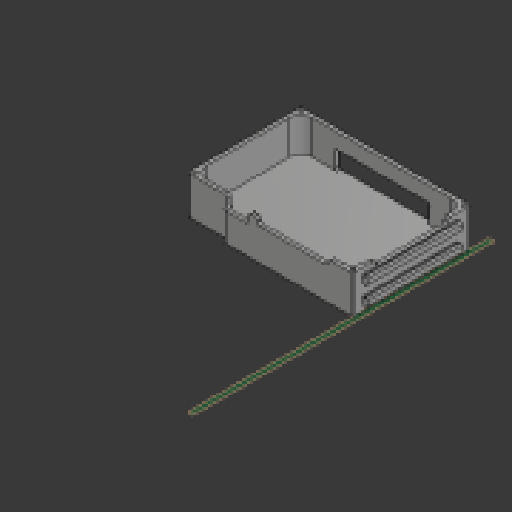
# Autodesk Inventor part: Back_Case
Saved by Autodesk Inventor 2023 (Build 270158000, 158)
## iProperties
Created: 2023-01-07
Part Number: Back_Case
Material: Generic
Document SubType Name: Modeling
Designer: alber
Density: 1 g/cm^3
Appearance: Smooth - Medium Gray
Author: alber
Autodesk Inventor part; units mm, degrees
ref_plane "YZ Plane" through (0, 0, 0) normal (1, 0, 0) x (0, 1, 0)
ref_plane "XZ Plane" through (0, 0, 0) normal (0, 1, 0) x (-1, 0, 0)
ref_plane "XY Plane" through (0, 0, 0) normal (0, 0, 1) x (1, 0, 0)
ref_plane "Work Plane1" through (64.9475, 0, 227.1619) normal (0, -1, 0) x (0, 0, 1)
sketch "Sketch1" plane through (64.9475, 0, 227.1619) normal (0, -1, 0) x (0, 0, 1)
  line L0 (-165, 215) -> (-165, 20) projected
  line L1 (-290, 20) -> (-165, 20)
  line L2 (-165, 20) -> (-165, 200)
  line L3 (-165, 200) -> (-290, 200)
  line L4 (-290, 200) -> (-290, 20)
  line L5 (0.8, 269) -> (0.8, 158) projected
  arc A0 (-0.2, 157) -> (0.8, 158) centre (-0.2, 158) ccw projected
  line L6 (-0.2, 157) -> (-164.2, 157) projected
  arc A1 (-165.2, 158) -> (-164.2, 157) centre (-164.2, 158) ccw projected
  line L7 (-165.2, 158) -> (-165.2, 269) projected
  arc A2 (-164.2, 270) -> (-165.2, 269) centre (-164.2, 269) ccw projected
  line L8 (-164.2, 270) -> (-126.2, 270) projected
  arc A3 (-125.2, 269) -> (-126.2, 270) centre (-126.2, 269) ccw projected
  line L9 (-125.2, 269) -> (-125.2, 267) projected
  arc A4 (-125.2, 267) -> (-124.2, 266) centre (-124.2, 267) ccw projected
  line L10 (-124.2, 266) -> (-116.2, 266) projected
  arc A5 (-116.2, 266) -> (-115.2, 267) centre (-116.2, 267) ccw projected
  line L11 (-115.2, 267) -> (-115.2, 269) projected
  arc A6 (-114.2, 270) -> (-115.2, 269) centre (-114.2, 269) ccw projected
  line L12 (-114.2, 270) -> (-0.2, 270) projected
  arc A7 (0.8, 269) -> (-0.2, 270) centre (-0.2, 269) ccw projected
  circle A8 centre (-38.2, 210.5) radius 5.1429 projected
  arc A9 (-20.2629, 212.0039) -> (-36.7039, 228.4377) centre (-38.2, 210.5) ccw projected
  line L13 (-36.7039, 228.4377) -> (-36.7039, 223.2698) projected
  arc A10 (-25.4311, 212.0039) -> (-36.7039, 223.2698) centre (-38.2, 210.5) ccw projected
  line L14 (-25.4311, 212.0039) -> (-20.2629, 212.0039) projected
  arc A11 (-28.0248, 212.0039) -> (-36.7039, 220.6763) centre (-38.2, 210.5) ccw projected
  line L15 (-36.7039, 220.6763) -> (-36.7039, 218.0678) projected
  arc A12 (-30.6322, 211.9961) -> (-36.7039, 218.0678) centre (-38.2, 210.5) ccw projected
  line L16 (-30.6322, 211.9961) -> (-30.6322, 212.0039) projected
  line L17 (-30.6322, 212.0039) -> (-28.0248, 212.0039) projected
  line L18 (-39.7039, 223.2689) -> (-39.7039, 228.4371) projected
  arc A13 (-39.7039, 228.4371) -> (-56.1377, 211.9961) centre (-38.2, 210.5) ccw projected
  line L19 (-56.1377, 211.9961) -> (-50.9698, 211.9961) projected
  arc A14 (-39.7039, 223.2689) -> (-50.9698, 211.9961) centre (-38.2, 210.5) ccw projected
  line L20 (-39.7039, 218.0678) -> (-39.7039, 220.6752) projected
  arc A15 (-39.7039, 220.6752) -> (-48.3763, 211.9961) centre (-38.2, 210.5) ccw projected
  line L21 (-48.3763, 211.9961) -> (-45.7678, 211.9961) projected
  arc A16 (-39.6961, 218.0678) -> (-45.7678, 211.9961) centre (-38.2, 210.5) ccw projected
  line L22 (-39.6961, 218.0678) -> (-39.7039, 218.0678) projected
  line L23 (-50.9689, 208.9961) -> (-56.1371, 208.9961) projected
  arc A17 (-56.1371, 208.9961) -> (-39.6961, 192.5623) centre (-38.2, 210.5) ccw projected
  line L24 (-39.6961, 192.5623) -> (-39.6961, 197.7302) projected
  arc A18 (-50.9689, 208.9961) -> (-39.6961, 197.7302) centre (-38.2, 210.5) ccw projected
  line L25 (-45.7678, 208.9961) -> (-48.3752, 208.9961) projected
  arc A19 (-48.3752, 208.9961) -> (-39.6961, 200.3237) centre (-38.2, 210.5) ccw projected
  line L26 (-39.6961, 200.3237) -> (-39.6961, 202.9322) projected
  arc A20 (-45.7678, 209.0039) -> (-39.6961, 202.9322) centre (-38.2, 210.5) ccw projected
  line L27 (-45.7678, 209.0039) -> (-45.7678, 208.9961) projected
  arc A21 (-36.6961, 197.7311) -> (-25.4302, 209.0039) centre (-38.2, 210.5) ccw projected
  line L28 (-36.6961, 197.7311) -> (-36.6961, 192.5629) projected
  arc A22 (-36.6961, 192.5629) -> (-20.2623, 209.0039) centre (-38.2, 210.5) ccw projected
  line L29 (-20.2623, 209.0039) -> (-25.4302, 209.0039) projected
  line L30 (-36.6961, 202.9322) -> (-36.6961, 200.3248) projected
  arc A23 (-36.6961, 200.3248) -> (-28.0237, 209.0039) centre (-38.2, 210.5) ccw projected
  line L31 (-28.0237, 209.0039) -> (-30.6322, 209.0039) projected
  arc A24 (-36.7039, 202.9322) -> (-30.6322, 209.0039) centre (-38.2, 210.5) ccw projected
  line L32 (-36.7039, 202.9322) -> (-36.6961, 202.9322) projected
  arc A25 (-137, 209.9) -> (-133.4, 209.9) centre (-135.2, 209.9) ccw projected
  line L33 (-133.4, 209.9) -> (-133.4, 214.1) projected
  arc A26 (-133.4, 214.1) -> (-137, 214.1) centre (-135.2, 214.1) ccw projected
  line L34 (-137, 214.1) -> (-137, 209.9) projected
  circle A27 centre (-6.7, 162) radius 2.1 projected
  circle A28 centre (-6.7, 265) radius 2.1 projected
  point P0 (-227.1619, 64.9475)
  point P1 (-165, 200)
  point P2 (-132.7045, 157)
  point P3 (-165.2, 200)
  point P4 (-165, 157.4)
  dimension "d0" = 125
  dimension "d1" = 180
  constraints: 8 end point, 2 parallel, 1 collinear, 1 horizontal, 1 perpendicular
  measures "d0" distance of L3.end L2.end
  measures "d1" distance of L2.end L1.end
extrude "Extrusion1" add sketch "Sketch1" against normal blind 4 contours L0 A1 L7 L3 | L0 L1 L4 L3 L7 A1
sketch "Sketch2" plane through (64.9475, 4, 227.1619) normal (0, 1, 0) x (1, 0, 0)
  line L0 (-20, 165) -> (-20, 290) projected
  line L1 (-20, 290) -> (-200, 290) projected
  line L2 (-200, 290) -> (-200, 165) projected
  line L3 (-200, 165) -> (-20, 165) projected
  line L4 (-24, 169) -> (-24, 286)
  line L5 (-24, 286) -> (-196, 286)
  line L6 (-196, 286) -> (-196, 169)
  line L7 (-196, 169) -> (-24, 169)
  arc A0 (-157, 164.2) -> (-158, 165.2) centre (-158, 164.2) ccw
  line L8 (-157, 160.2816) -> (-157, 164.2)
  line L9 (-158, 165.2) -> (-196, 165.2)
  line L10 (-200, 165.2) -> (-269, 165.2)
  line L11 (-153, 164.2) -> (-153, 160.2816)
  point P0 (-64.9475, 227.1619)
  point P1 (-157.0033, 164.2816)
  dimension "d4" = 4
  constraints: 16 end point, 2 horizontal, 2 point on circle, 2 point on line, 1 centre point, 1 vertical, 11 other
ref_plane "Work Plane2" through (45.1475, 40, -62.8381) normal (0, 1, 0) x (0, 0, 1)
extrude "Extrusion2" add sketch "Sketch2" along normal up to surface (36 mm away)
sketch "Sketch3" plane through (44.9475, 0, -62.8381) normal (0, 0, -1) x (-1, 0, 0)
  line L0 (-25.1172, 40) -> (-14.8828, 40) projected
  arc A0 (-25.1172, 40) -> (-25.2586, 39.9414) centre (-25.1172, 39.8) ccw projected
  line L1 (-26.6586, 38.5414) -> (-25.2586, 39.9414) projected
  arc A1 (-26.6586, 38.5414) -> (-26.5172, 38.2) centre (-26.5172, 38.4) ccw projected
  line L2 (-26.5172, 38.2) -> (-24.7899, 38.2) projected
  line L3 (-24.7899, 36.2) -> (-24.7899, 38.2) projected
  line L4 (-26.9899, 34) -> (-24.7899, 36.2) projected
  line L5 (-29.5, 34) -> (-26.9899, 34) projected
  line L6 (-29.5, 34) -> (-30, 33.5) projected
  line L7 (-30, 33.5) -> (-30.5, 34) projected
  line L8 (-33.0101, 34) -> (-30.5, 34) projected
  line L9 (-35.2101, 36.2) -> (-33.0101, 34) projected
  line L10 (-35.2101, 38.2) -> (-35.2101, 36.2) projected
  line L11 (-35.2101, 38.2) -> (-33.4828, 38.2) projected
  arc A2 (-33.4828, 38.2) -> (-33.3414, 38.5414) centre (-33.4828, 38.4) ccw projected
  line L12 (-34.7414, 39.9414) -> (-33.3414, 38.5414) projected
  arc A3 (-34.7414, 39.9414) -> (-34.8828, 40) centre (-34.8828, 39.8) ccw projected
  line L13 (-39.8, 40) -> (-34.8828, 40) projected
  arc A4 (-39.8, 40) -> (-40, 39.8) centre (-39.8, 39.8) ccw projected
  line L14 (-40, 34.8828) -> (-40, 39.8) projected
  arc A5 (-40, 34.8828) -> (-39.9414, 34.7414) centre (-39.8, 34.8828) ccw projected
  line L15 (-38.5414, 33.3414) -> (-39.9414, 34.7414) projected
  arc A6 (-38.5414, 33.3414) -> (-38.2, 33.4828) centre (-38.4, 33.4828) ccw projected
  line L16 (-38.2, 33.4828) -> (-38.2, 35.2101) projected
  line L17 (-36.2, 35.2101) -> (-38.2, 35.2101) projected
  line L18 (-34, 33.0101) -> (-36.2, 35.2101) projected
  line L19 (-34, 30.5) -> (-34, 33.0101) projected
  line L20 (-34, 30.5) -> (-33.5, 30) projected
  line L21 (-33.5, 30) -> (-34, 29.5) projected
  line L22 (-34, 26.9899) -> (-34, 29.5) projected
  line L23 (-36.2, 24.7899) -> (-34, 26.9899) projected
  line L24 (-38.2, 24.7899) -> (-36.2, 24.7899) projected
  line L25 (-38.2, 24.7899) -> (-38.2, 26.5172) projected
  arc A7 (-38.2, 26.5172) -> (-38.5414, 26.6586) centre (-38.4, 26.5172) ccw projected
  line L26 (-39.9414, 25.2586) -> (-38.5414, 26.6586) projected
  arc A8 (-39.9414, 25.2586) -> (-40, 25.1172) centre (-39.8, 25.1172) ccw projected
  line L27 (-40, 14.8) -> (-40, 25.1172) projected
  line L28 (-38.2, 13) -> (-40, 14.8) projected
  line L29 (-38.2, 15.2101) -> (-38.2, 13) projected
  line L30 (-36.2, 15.2101) -> (-38.2, 15.2101) projected
  line L31 (-34, 13.0101) -> (-36.2, 15.2101) projected
  line L32 (-34, 10.5) -> (-34, 13.0101) projected
  line L33 (-33.5, 10) -> (-34, 10.5) projected
  line L34 (-34, 9.5) -> (-33.5, 10) projected
  line L35 (-34, 6.9899) -> (-34, 9.5) projected
  line L36 (-36.2, 4.7899) -> (-34, 6.9899) projected
  line L37 (-38.2, 4.7899) -> (-36.2, 4.7899) projected
  line L38 (-38.2, 7) -> (-38.2, 4.7899) projected
  line L39 (-40, 5.2) -> (-38.2, 7) projected
  line L40 (-40, 0) -> (-40, 5.2) projected
  line L41 (-34.8, 0) -> (-40, 0) projected
  line L42 (-33, 1.8) -> (-34.8, 0) projected
  line L43 (-35.2101, 1.8) -> (-33, 1.8) projected
  line L44 (-35.2101, 3.8) -> (-35.2101, 1.8) projected
  line L45 (-33.0101, 6) -> (-35.2101, 3.8) projected
  line L46 (-30.5, 6) -> (-33.0101, 6) projected
  line L47 (-30, 6.5) -> (-30.5, 6) projected
  line L48 (-29.5, 6) -> (-30, 6.5) projected
  line L49 (-26.9899, 6) -> (-29.5, 6) projected
  line L50 (-24.7899, 3.8) -> (-26.9899, 6) projected
  line L51 (-24.7899, 1.8) -> (-24.7899, 3.8) projected
  line L52 (-27, 1.8) -> (-24.7899, 1.8) projected
  line L53 (-25.2, 0) -> (-27, 1.8) projected
  line L54 (-14.8, 0) -> (-25.2, 0) projected
  line L55 (-13, 1.8) -> (-14.8, 0) projected
  line L56 (-15.2101, 1.8) -> (-13, 1.8) projected
  line L57 (-15.2101, 3.8) -> (-15.2101, 1.8) projected
  line L58 (-13.0101, 6) -> (-15.2101, 3.8) projected
  line L59 (-10.5, 6) -> (-13.0101, 6) projected
  line L60 (-10, 6.5) -> (-10.5, 6) projected
  line L61 (-9.5, 6) -> (-10, 6.5) projected
  line L62 (-6.9899, 6) -> (-9.5, 6) projected
  line L63 (-4.7899, 3.8) -> (-6.9899, 6) projected
  line L64 (-4.7899, 1.8) -> (-4.7899, 3.8) projected
  line L65 (-7, 1.8) -> (-4.7899, 1.8) projected
  line L66 (-5.2, 0) -> (-7, 1.8) projected
  line L67 (0, 0) -> (-5.2, 0) projected
  line L68 (0, 5.2) -> (0, 0) projected
  line L69 (-1.8, 7) -> (0, 5.2) projected
  line L70 (-1.8, 4.7899) -> (-1.8, 7) projected
  line L71 (-3.8, 4.7899) -> (-1.8, 4.7899) projected
  line L72 (-6, 6.9899) -> (-3.8, 4.7899) projected
  line L73 (-6, 9.5) -> (-6, 6.9899) projected
  line L74 (-6.5, 10) -> (-6, 9.5) projected
  line L75 (-6, 10.5) -> (-6.5, 10) projected
  line L76 (-6, 13.0101) -> (-6, 10.5) projected
  line L77 (-3.8, 15.2101) -> (-6, 13.0101) projected
  line L78 (-1.8, 15.2101) -> (-3.8, 15.2101) projected
  line L79 (-1.8, 13) -> (-1.8, 15.2101) projected
  line L80 (0, 14.8) -> (-1.8, 13) projected
  line L81 (0, 25.1172) -> (0, 14.8) projected
  arc A9 (0, 25.1172) -> (-0.0586, 25.2586) centre (-0.2, 25.1172) ccw projected
  line L82 (-1.4586, 26.6586) -> (-0.0586, 25.2586) projected
  arc A10 (-1.4586, 26.6586) -> (-1.8, 26.5172) centre (-1.6, 26.5172) ccw projected
  line L83 (-1.8, 26.5172) -> (-1.8, 24.7899) projected
  line L84 (-3.8, 24.7899) -> (-1.8, 24.7899) projected
  line L85 (-6, 26.9899) -> (-3.8, 24.7899) projected
  line L86 (-6, 29.5) -> (-6, 26.9899) projected
  line L87 (-6, 29.5) -> (-6.5, 30) projected
  line L88 (-6.5, 30) -> (-6, 30.5) projected
  line L89 (-6, 33.0101) -> (-6, 30.5) projected
  line L90 (-3.8, 35.2101) -> (-6, 33.0101) projected
  line L91 (-1.8, 35.2101) -> (-3.8, 35.2101) projected
  line L92 (-1.8, 35.2101) -> (-1.8, 33.4828) projected
  arc A11 (-1.8, 33.4828) -> (-1.4586, 33.3414) centre (-1.6, 33.4828) ccw projected
  line L93 (-0.0586, 34.7414) -> (-1.4586, 33.3414) projected
  arc A12 (-0.0586, 34.7414) -> (0, 34.8828) centre (-0.2, 34.8828) ccw projected
  line L94 (0, 39.8) -> (0, 34.8828) projected
  arc A13 (0, 39.8) -> (-0.2, 40) centre (-0.2, 39.8) ccw projected
  line L95 (-5.1172, 40) -> (-0.2, 40) projected
  arc A14 (-5.1172, 40) -> (-5.2586, 39.9414) centre (-5.1172, 39.8) ccw projected
  line L96 (-6.6586, 38.5414) -> (-5.2586, 39.9414) projected
  arc A15 (-6.6586, 38.5414) -> (-6.5172, 38.2) centre (-6.5172, 38.4) ccw projected
  line L97 (-6.5172, 38.2) -> (-4.7899, 38.2) projected
  line L98 (-4.7899, 36.2) -> (-4.7899, 38.2) projected
  line L99 (-6.9899, 34) -> (-4.7899, 36.2) projected
  line L100 (-9.5, 34) -> (-6.9899, 34) projected
  line L101 (-9.5, 34) -> (-10, 33.5) projected
  line L102 (-10, 33.5) -> (-10.5, 34) projected
  line L103 (-13.0101, 34) -> (-10.5, 34) projected
  line L104 (-15.2101, 36.2) -> (-13.0101, 34) projected
  line L105 (-15.2101, 38.2) -> (-15.2101, 36.2) projected
  line L106 (-15.2101, 38.2) -> (-13.4828, 38.2) projected
  arc A16 (-13.4828, 38.2) -> (-13.3414, 38.5414) centre (-13.4828, 38.4) ccw projected
  line L107 (-14.7414, 39.9414) -> (-13.3414, 38.5414) projected
  arc A17 (-14.7414, 39.9414) -> (-14.8828, 40) centre (-14.8828, 39.8) ccw projected
  circle A18 centre (-30, 30) radius 3 projected
  circle A19 centre (-10, 10) radius 3 projected
  circle A20 centre (-10, 30) radius 2.5 projected
  circle A21 centre (-30, 10) radius 2.5 projected
  line L108 (-13.0101, 14) -> (-14, 13.0101) projected
  line L109 (-14, 10.5) -> (-14, 13.0101) projected
  line L110 (-13.5, 10) -> (-14, 10.5) projected
  line L111 (-14, 9.5) -> (-13.5, 10) projected
  line L112 (-14, 6.9899) -> (-14, 9.5) projected
  line L113 (-16.2, 4.7899) -> (-14, 6.9899) projected
  line L114 (-23.8, 4.7899) -> (-16.2, 4.7899) projected
  line L115 (-26, 6.9899) -> (-23.8, 4.7899) projected
  line L116 (-26, 9.5) -> (-26, 6.9899) projected
  line L117 (-26.5, 10) -> (-26, 9.5) projected
  line L118 (-26, 10.5) -> (-26.5, 10) projected
  line L119 (-26, 13.0101) -> (-26, 10.5) projected
  line L120 (-26, 13.0101) -> (-26.9899, 14) projected
  line L121 (-29.5, 14) -> (-26.9899, 14) projected
  line L122 (-30, 13.5) -> (-29.5, 14) projected
  line L123 (-30.5, 14) -> (-30, 13.5) projected
  line L124 (-33.0101, 14) -> (-30.5, 14) projected
  line L125 (-35.2101, 16.2) -> (-33.0101, 14) projected
  line L126 (-38.2, 16.2) -> (-35.2101, 16.2) projected
  line L127 (-38.2, 23.8) -> (-38.2, 16.2) projected
  line L128 (-35.2101, 23.8) -> (-38.2, 23.8) projected
  line L129 (-33.0101, 26) -> (-35.2101, 23.8) projected
  line L130 (-30.5, 26) -> (-33.0101, 26) projected
  line L131 (-30.5, 26) -> (-30, 26.5) projected
  line L132 (-30, 26.5) -> (-29.5, 26) projected
  line L133 (-26.9899, 26) -> (-29.5, 26) projected
  line L134 (-26.9899, 26) -> (-26, 26.9899) projected
  line L135 (-26, 29.5) -> (-26, 26.9899) projected
  line L136 (-26, 29.5) -> (-26.5, 30) projected
  line L137 (-26.5, 30) -> (-26, 30.5) projected
  line L138 (-26, 33.0101) -> (-26, 30.5) projected
  line L139 (-23.8, 35.2101) -> (-26, 33.0101) projected
  line L140 (-16.2, 35.2101) -> (-23.8, 35.2101) projected
  line L141 (-14, 33.0101) -> (-16.2, 35.2101) projected
  line L142 (-14, 30.5) -> (-14, 33.0101) projected
  line L143 (-14, 30.5) -> (-13.5, 30) projected
  line L144 (-13.5, 30) -> (-14, 29.5) projected
  line L145 (-14, 26.9899) -> (-14, 29.5) projected
  line L146 (-14, 26.9899) -> (-13.0101, 26) projected
  line L147 (-10.5, 26) -> (-13.0101, 26) projected
  line L148 (-10.5, 26) -> (-10, 26.5) projected
  line L149 (-10, 26.5) -> (-9.5, 26) projected
  line L150 (-6.9899, 26) -> (-9.5, 26) projected
  line L151 (-4.7899, 23.8) -> (-6.9899, 26) projected
  line L152 (-1.8, 23.8) -> (-4.7899, 23.8) projected
  line L153 (-1.8, 16.2) -> (-1.8, 23.8) projected
  line L154 (-4.7899, 16.2) -> (-1.8, 16.2) projected
  line L155 (-6.9899, 14) -> (-4.7899, 16.2) projected
  line L156 (-9.5, 14) -> (-6.9899, 14) projected
  line L157 (-10, 13.5) -> (-9.5, 14) projected
  line L158 (-10.5, 14) -> (-10, 13.5) projected
  line L159 (-13.0101, 14) -> (-10.5, 14) projected
  line L160 (0, 0) -> (0, 40) projected
  line L161 (-5.6, 32.8444) -> (-5.6, 30.3343)
  line L162 (-5.6, 30.3343) -> (-5.9343, 30)
  line L163 (-5.9343, 30) -> (-5.6, 29.6657)
  line L164 (-5.6, 29.6657) -> (-5.6, 27.1556)
  line L165 (-5.6, 27.1556) -> (-3.6343, 25.1899)
  line L166 (-3.6343, 25.1899) -> (-2.2, 25.1899)
  line L167 (-2.2, 25.1899) -> (-2.2, 26.5172)
  arc A22 (-1.1757, 26.9414) -> (-2.2, 26.5172) centre (-1.6, 26.5172) ccw
  line L168 (-1.1757, 26.9414) -> (0.2243, 25.5414)
  arc A23 (0.4, 25.1172) -> (0.2243, 25.5414) centre (-0.2, 25.1172) ccw
  line L169 (0.4, 25.1172) -> (0.4, 14.6343)
  line L170 (0.4, 14.6343) -> (-1.1757, 13.0586)
  line L171 (-2.2, 13.4828) -> (-2.2, 14.8101)
  line L172 (-2.2, 14.8101) -> (-3.6343, 14.8101)
  line L173 (-3.6343, 14.8101) -> (-5.6, 12.8444)
  line L174 (-5.6, 12.8444) -> (-5.6, 10.3343)
  line L175 (-5.6, 10.3343) -> (-5.9343, 10)
  line L176 (-5.9343, 10) -> (-5.6, 9.6657)
  line L177 (-5.6, 9.6657) -> (-5.6, 7.1556)
  line L178 (-5.6, 7.1556) -> (-3.6343, 5.1899)
  line L179 (-3.6343, 5.1899) -> (-2.2, 5.1899)
  line L180 (-2.2, 5.1899) -> (-2.2, 6.5172)
  line L181 (-1.1757, 6.9414) -> (0.4, 5.3657)
  line L182 (0.4, 5.3657) -> (0.4, -0.4)
  line L183 (0.4, -0.4) -> (-5.3657, -0.4)
  line L184 (-5.3657, -0.4) -> (-7.9657, 2.2)
  line L185 (-7.9657, 2.2) -> (-5.1899, 2.2)
  line L186 (-5.1899, 2.2) -> (-5.1899, 3.6343)
  line L187 (-5.1899, 3.6343) -> (-7.1556, 5.6)
  line L188 (-7.1556, 5.6) -> (-9.6657, 5.6)
  line L189 (-9.6657, 5.6) -> (-10, 5.9343)
  line L190 (-10, 5.9343) -> (-10.3343, 5.6)
  line L191 (-10.3343, 5.6) -> (-12.8444, 5.6)
  line L192 (-12.8444, 5.6) -> (-14.8101, 3.6343)
  line L193 (-14.8101, 3.6343) -> (-14.8101, 2.2)
  line L194 (-14.8101, 2.2) -> (-12.0343, 2.2)
  line L195 (-12.0343, 2.2) -> (-14.6343, -0.4)
  line L196 (-14.6343, -0.4) -> (-25.3657, -0.4)
  line L197 (-25.3657, -0.4) -> (-27.9657, 2.2)
  line L198 (-27.9657, 2.2) -> (-25.1899, 2.2)
  line L199 (-25.1899, 2.2) -> (-25.1899, 3.6343)
  line L200 (-25.1899, 3.6343) -> (-27.1556, 5.6)
  line L201 (-27.1556, 5.6) -> (-29.6657, 5.6)
  line L202 (-29.6657, 5.6) -> (-30, 5.9343)
  line L203 (-30, 5.9343) -> (-30.3343, 5.6)
  line L204 (-30.3343, 5.6) -> (-32.8444, 5.6)
  line L205 (-32.8444, 5.6) -> (-34.8101, 3.6343)
  line L206 (-34.8101, 3.6343) -> (-34.8101, 2.2)
  line L207 (-34.8101, 2.2) -> (-32.0343, 2.2)
  line L208 (-32.0343, 2.2) -> (-34.6343, -0.4)
  line L209 (-34.6343, -0.4) -> (-40.4, -0.4)
  line L210 (-40.4, -0.4) -> (-40.4, 5.3657)
  line L211 (-40.4, 5.3657) -> (-37.8, 7.9657)
  line L212 (-37.8, 7.9657) -> (-37.8, 5.1899)
  line L213 (-37.8, 5.1899) -> (-36.3657, 5.1899)
  line L214 (-36.3657, 5.1899) -> (-34.4, 7.1556)
  line L215 (-34.4, 7.1556) -> (-34.4, 9.6657)
  line L216 (-34.4, 9.6657) -> (-34.0657, 10)
  line L217 (-34.0657, 10) -> (-34.4, 10.3343)
  line L218 (-34.4, 10.3343) -> (-34.4, 12.8444)
  line L219 (-34.4, 12.8444) -> (-36.3657, 14.8101)
  line L220 (-36.3657, 14.8101) -> (-37.8, 14.8101)
  line L221 (-37.8, 14.8101) -> (-37.8, 12.0343)
  line L222 (-37.8, 12.0343) -> (-40.4, 14.6343)
  line L223 (-40.4, 14.6343) -> (-40.4, 25.1172)
  arc A24 (-40.2243, 25.5414) -> (-40.4, 25.1172) centre (-39.8, 25.1172) ccw
  line L224 (-40.2243, 25.5414) -> (-38.8243, 26.9414)
  arc A25 (-37.8, 26.5172) -> (-38.8243, 26.9414) centre (-38.4, 26.5172) ccw
  line L225 (-37.8, 26.5172) -> (-37.8, 25.1899)
  line L226 (-37.8, 25.1899) -> (-36.3657, 25.1899)
  line L227 (-36.3657, 25.1899) -> (-34.4, 27.1556)
  line L228 (-34.4, 27.1556) -> (-34.4, 29.6657)
  line L229 (-34.4, 29.6657) -> (-34.0657, 30)
  line L230 (-34.0657, 30) -> (-34.4, 30.3343)
  line L231 (-34.4, 30.3343) -> (-34.4, 32.8444)
  line L232 (-34.4, 32.8444) -> (-36.3657, 34.8101)
  line L233 (-36.3657, 34.8101) -> (-37.8, 34.8101)
  line L234 (-37.8, 34.8101) -> (-37.8, 33.4828)
  arc A26 (-38.8243, 33.0586) -> (-37.8, 33.4828) centre (-38.4, 33.4828) ccw
  line L235 (-38.8243, 33.0586) -> (-40.2243, 34.4586)
  arc A27 (-40.4, 34.8828) -> (-40.2243, 34.4586) centre (-39.8, 34.8828) ccw
  line L236 (-40.4, 34.8828) -> (-40.4, 39.8)
  arc A28 (-39.8, 40.4) -> (-40.4, 39.8) centre (-39.8, 39.8) ccw
  line L237 (-39.8, 40.4) -> (-34.8828, 40.4)
  arc A29 (-34.4586, 40.2243) -> (-34.8828, 40.4) centre (-34.8828, 39.8) ccw
  line L238 (-34.4586, 40.2243) -> (-33.0586, 38.8243)
  arc A30 (-33.4828, 37.8) -> (-33.0586, 38.8243) centre (-33.4828, 38.4) ccw
  line L239 (-33.4828, 37.8) -> (-34.8101, 37.8)
  line L240 (-34.8101, 37.8) -> (-34.8101, 36.3657)
  line L241 (-34.8101, 36.3657) -> (-32.8444, 34.4)
  line L242 (-32.8444, 34.4) -> (-30.3343, 34.4)
  line L243 (-30.3343, 34.4) -> (-30, 34.0657)
  line L244 (-30, 34.0657) -> (-29.6657, 34.4)
  line L245 (-29.6657, 34.4) -> (-27.1556, 34.4)
  line L246 (-27.1556, 34.4) -> (-25.1899, 36.3657)
  line L247 (-25.1899, 36.3657) -> (-25.1899, 37.8)
  line L248 (-25.1899, 37.8) -> (-26.5172, 37.8)
  arc A31 (-26.9414, 38.8243) -> (-26.5172, 37.8) centre (-26.5172, 38.4) ccw
  line L249 (-26.9414, 38.8243) -> (-25.5414, 40.2243)
  arc A32 (-25.1172, 40.4) -> (-25.5414, 40.2243) centre (-25.1172, 39.8) ccw
  line L250 (-25.1172, 40.4) -> (-14.8828, 40.4)
  arc A33 (-14.4586, 40.2243) -> (-14.8828, 40.4) centre (-14.8828, 39.8) ccw
  line L251 (-14.4586, 40.2243) -> (-13.0586, 38.8243)
  arc A34 (-13.4828, 37.8) -> (-13.0586, 38.8243) centre (-13.4828, 38.4) ccw
  line L252 (-13.4828, 37.8) -> (-14.8101, 37.8)
  line L253 (-14.8101, 37.8) -> (-14.8101, 36.3657)
  line L254 (-14.8101, 36.3657) -> (-12.8444, 34.4)
  line L255 (-12.8444, 34.4) -> (-10.3343, 34.4)
  line L256 (-10.3343, 34.4) -> (-10, 34.0657)
  line L257 (-10, 34.0657) -> (-9.6657, 34.4)
  line L258 (-9.6657, 34.4) -> (-7.1556, 34.4)
  line L259 (-7.1556, 34.4) -> (-5.1899, 36.3657)
  line L260 (-5.1899, 36.3657) -> (-5.1899, 37.8)
  line L261 (-5.1899, 37.8) -> (-6.5172, 37.8)
  arc A35 (-6.9414, 38.8243) -> (-6.5172, 37.8) centre (-6.5172, 38.4) ccw
  line L262 (-6.9414, 38.8243) -> (-5.5414, 40.2243)
  arc A36 (-5.1172, 40.4) -> (-5.5414, 40.2243) centre (-5.1172, 39.8) ccw
  line L263 (-5.1172, 40.4) -> (-0.2, 40.4)
  arc A37 (0.4, 39.8) -> (-0.2, 40.4) centre (-0.2, 39.8) ccw
  line L264 (0.4, 39.8) -> (0.4, 34.8828)
  arc A38 (0.2243, 34.4586) -> (0.4, 34.8828) centre (-0.2, 34.8828) ccw
  line L265 (0.2243, 34.4586) -> (-1.1757, 33.0586)
  arc A39 (-2.2, 33.4828) -> (-1.1757, 33.0586) centre (-1.6, 33.4828) ccw
  line L266 (-2.2, 33.4828) -> (-2.2, 34.8101)
  line L267 (-2.2, 34.8101) -> (-3.6343, 34.8101)
  line L268 (-3.6343, 34.8101) -> (-5.6, 32.8444)
  arc A40 (-2.2, 13.4828) -> (-1.1757, 13.0586) centre (-1.6, 13.4828) ccw
  arc A41 (-1.1757, 6.9414) -> (-2.2, 6.5172) centre (-1.6, 6.5172) ccw
  line L269 (-5.6, 10.3343) -> (-5.6, 9.6657)
  line L270 (-5.6, 30.3343) -> (-5.6, 29.6657)
  point P0 (44.9475, 0)
  point P1 (0, 25.7657)
  point P2 (0, 34.2343)
  point P3 (0, 5.7657)
  point P4 (0, 14.2343)
  point P5 (0, 4)
  dimension "d7" = 0.4
  dimension "d8" = 0.6
  dimension "d9" = 0.6
  constraints: 220 end point, 40 point on circle, 20 centre point, 4 tangent, 1 collinear, 1 vertical, 125 other
  measures "d7" distance between parallel lines of L90 L268
  measures "d8" radius of A40
  measures "d9" radius of A41
extrude "Extrusion3" add sketch "Sketch3" against normal blind 115 contours L160 L168 A22 L167 L166 L165 L164 L270 L161 L268 L267 L266 A39 L265 | L160 L181 A41 L180 L179 L178 L177 L269 L174 L173 L172 L171 A40 L170
sketch "Sketch4" plane through (44.9475, 0, -62.8381) normal (0, 0, -1) x (-1, 0, 0)
  line L0 (180, 0) -> (0, 0) projected
  line L1 (180, 0) -> (180, 40) projected
  line L2 (0, 34.2343) -> (0, 40) projected
  line L3 (0, 25.7657) -> (0, 34.2343) projected
  line L4 (0, 5.7657) -> (0, 34.2343)
  line L5 (180, 40) -> (0, 40) projected
  line L6 (0, 34.2343) -> (-1.1757, 33.0586) projected
  arc A0 (-2.2, 33.4828) -> (-1.1757, 33.0586) centre (-1.6, 33.4828) ccw projected
  line L7 (-2.2, 33.4828) -> (-2.2, 34.8101) projected
  line L8 (-2.2, 34.8101) -> (-3.6343, 34.8101) projected
  line L9 (-3.6343, 34.8101) -> (-5.6, 32.8444) projected
  line L10 (-5.6, 32.8444) -> (-5.6, 27.1556) projected
  line L11 (-5.6, 27.1556) -> (-3.6343, 25.1899) projected
  line L12 (-3.6343, 25.1899) -> (-2.2, 25.1899) projected
  line L13 (-2.2, 25.1899) -> (-2.2, 26.5172) projected
  arc A1 (-1.1757, 26.9414) -> (-2.2, 26.5172) centre (-1.6, 26.5172) ccw projected
  line L14 (-1.1757, 26.9414) -> (0, 25.7657) projected
  line L15 (0, 14.2343) -> (0, 25.7657) projected
  line L16 (0, 14.2343) -> (-1.1757, 13.0586) projected
  arc A2 (-2.2, 13.4828) -> (-1.1757, 13.0586) centre (-1.6, 13.4828) ccw projected
  line L17 (-2.2, 13.4828) -> (-2.2, 14.8101) projected
  line L18 (-2.2, 14.8101) -> (-3.6343, 14.8101) projected
  line L19 (-3.6343, 14.8101) -> (-5.6, 12.8444) projected
  line L20 (-5.6, 12.8444) -> (-5.6, 7.1556) projected
  line L21 (-5.6, 7.1556) -> (-3.6343, 5.1899) projected
  line L22 (-3.6343, 5.1899) -> (-2.2, 5.1899) projected
  line L23 (-2.2, 5.1899) -> (-2.2, 6.5172) projected
  arc A3 (-1.1757, 6.9414) -> (-2.2, 6.5172) centre (-1.6, 6.5172) ccw projected
  line L24 (-1.1757, 6.9414) -> (0, 5.7657) projected
  line L25 (0, 0) -> (0, 5.7657) projected
  point P0 (44.9475, 0)
  point P1 (0, 14.2343)
  point P2 (0, 34.2343)
  point P3 (0, 25.7657)
  constraints: 2 end point
extrude "Extrusion4" cut sketch "Sketch4" against normal blind 15 contours L24 A3 L23 L22 L21 L20 L19 L18 L17 A2 L16 L4 | L3 L14 A1 L13 L12 L11 L10 L9 L8 L7 A0 L6
fillet "Fillet1" radius 2 4 edges at (-135.0525, 20, -62.8381) (44.9475, 20, -62.8381) (44.9475, 20, 62.1619) (-135.0525, 20, 62.1619)
fillet "Fillet2" radius 12 4 edges at (40.9475, 22, 58.1619) (40.9475, 22, -58.8381) (-131.0525, 22, -58.8381) (-131.0525, 22, 58.1619)
sketch "Sketch6" plane through (40.9475, 4, -46.8381) normal (-1, 0, 0) x (0, 0, 1)
  line L0 (93, 36) -> (0, 36) projected
  line L1 (9, 36) -> (84, 36)
  line L2 (84, 36) -> (84, 30)
  line L3 (84, 30) -> (9, 30)
  line L4 (9, 30) -> (9, 36)
  line L5 (0, 0) -> (0, 36) projected
  line L6 (93, 36) -> (93, 0) projected
  point P0 (46.8381, -4)
  point P1 (84, 36)
  dimension "d22" = 75
  dimension "d23" = 6
  dimension "d24" = 93
  dimension "d25" = 9
  constraints: 8 end point, 2 parallel, 1 horizontal, 1 perpendicular, 1 point on line
  measures "d22" distance of L2.end L3.end
  measures "d23" distance of L1.end L2.end
  measures "d24" distance between parallel lines of L5 L6
  measures "d25" distance between parallel lines of L5 L4
extrude "Extrusion6" cut sketch "Sketch6" against normal blind 6
fillet "Fillet3" radius 3 4 edges at (43.0647, 34, 37.1619) (42.9475, 40, 37.1619) (42.9475, 40, -37.8381) (43.0647, 34, -37.8381)
sketch "Sketch7" plane through (28.9475, 4, 58.1619) normal (0, 0, -1) x (-1, 0, 0)
  line L0 (-14, 36) -> (162, 36) projected
  line L1 (10.0678, 36) -> (85.0678, 36)
  line L2 (85.0678, 36) -> (85.0678, 30)
  line L3 (85.0678, 30) -> (10.0678, 30)
  line L4 (10.0678, 30) -> (10.0678, 36)
  line L5 (99, 30.8) -> (99, 36) projected
  line L6 (0, 0) -> (0, 36) projected
  point P0 (28.9475, -4)
  point P1 (85.0678, 36)
  point P2 (121, 36)
  point P3 (119, 36)
  dimension "d29" = 75
  dimension "d30" = 6
  dimension "d31" = 95.1355
  dimension "d32" = 10.0678
  constraints: 8 end point, 2 parallel, 1 horizontal, 1 perpendicular, 1 point on line
  measures "d29" distance of L2.end L3.end
  measures "d30" distance of L1.end L2.end
  measures "d32" distance between parallel lines of L6 L4
extrude "Extrusion7" cut sketch "Sketch7" against normal blind 10.5
fillet "Fillet4" radius 3 4 edges at (-56.1202, 40, 60.1619) (-56.1202, 34, 60.1619) (18.8798, 40, 60.1619) (18.8798, 34, 60.1619)
sketch "Sketch11" plane through (28.9475, 4, 58.1619) normal (0, 0, -1) x (-1, 0, 0)
  line L0 (148, 36) -> (88.0678, 36) projected
  line L1 (124.9086, 36) -> (74.9086, 36)
  line L2 (74.9086, 36) -> (74.9086, 26)
  line L3 (74.9086, 26) -> (124.9086, 26)
  line L4 (124.9086, 26) -> (124.9086, 36)
  point P0 (28.9475, -4)
  dimension "d56" = 50
  dimension "d57" = 10
  constraints: 8 end point, 2 parallel, 1 horizontal, 1 perpendicular, 1 point on line
  measures "d56" distance of L3.end L2.end
  measures "d57" distance of L1.end L2.end
extrude "Extrusion11" cut sketch "Sketch11" against normal blind 23
fillet "Fillet7" radius 3 4 edges at (-45.9611, 34, 60.1619) (-45.9611, 30, 60.1619) (-95.9611, 30, 60.1619) (-95.9611, 40, 60.1619)
equation "\"d25\" = -0.5 * d22 + 0.5 * d24"
equation "\"d32\" = -0.5 * d29 + 0.5 * d31"
body "Solid1"
